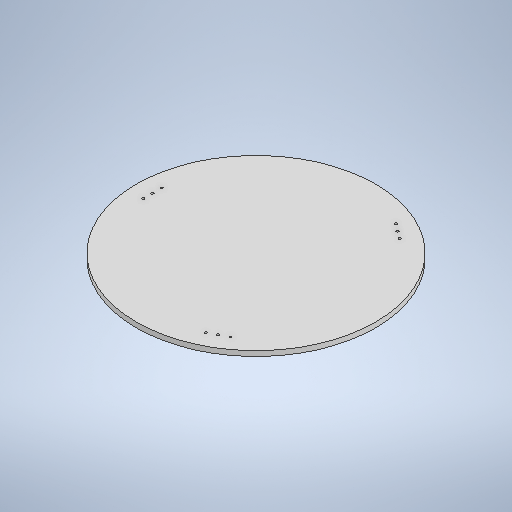
# Autodesk Inventor part: plate support
Saved by Autodesk Inventor 2025.1 (Build 291241000, 241)
## iProperties
Created: 2024-10-31
Part Number: plate support
Material: Generic
Document SubType Name: Modeling
Designer: xingj
Density: 1 g/cm^3
Appearance: Default
Author: xingj
Autodesk Inventor part; units mm, degrees
ref_plane "YZ Plane" through (0, 0, 0) normal (1, 0, 0) x (0, 1, 0)
ref_plane "XZ Plane" through (0, 0, 0) normal (0, 1, 0) x (-1, 0, 0)
ref_plane "XY Plane" through (0, 0, 0) normal (0, 0, 1) x (1, 0, 0)
sketch "Sketch1" plane through (0, 0, 0) normal (0, 1, 0) x (-1, 0, 0)
  circle A0 centre (0, 0) radius 150
  line L0 (150, 0) -> (0, 0)
  line L1 (0, 0) -> (-75, -129.9038)
  line L2 (0, 0) -> (150, 0) construction
  line L3 (0, 0) -> (-75, 129.9038)
  line L4 (0, 0) -> (150, 0) construction
  line L5 (-75, 129.9038) -> (-74.5, 129.0378)
  line L6 (-74.5, 129.0378) -> (-69.335, 120.0917)
  line L7 (-75, 129.9038) -> (-64.967, 112.5261)
  circle A1 centre (-64.967, 112.5261) radius 1.5
  line L8 (150, 0) -> (129.934, 0)
  circle A2 centre (129.934, 0) radius 1.5
  line L9 (-75, -129.9038) -> (-64.967, -112.5261)
  circle A3 centre (-64.967, -112.5261) radius 1.5
  dimension "d20" = 300
  dimension "d22" = 120
  dimension "d23" = 120
  dimension "d24" = 1
  dimension "d25" = 10.33
  dimension "d26" = 20.066
  dimension "d27" = 3
  dimension "d28" = 20.066
  dimension "d29" = 3
  dimension "d30" = 20.066
  dimension "d31" = 3
  constraints: 20 end point, 5 coincident, 5 point on line, 4 centre point, 3 horizontal, 3 point on circle, 2 equal length
  measures "d20" diameter of A0
  measures "d22" angle of L1 L2
  measures "d23" angle of L4 L3
  measures "d24" distance of L3.end L5.end
  measures "d25" distance of L5.end L6.end
  measures "d26" distance of L3.end L7.end
  measures "d27" diameter of A1
  measures "d28" distance of L4.end L8.end
  measures "d29" diameter of A2
  measures "d30" distance of L1.end L9.end
  measures "d31" diameter of A3
extrude "Extrusion1" add sketch "Sketch1" along normal blind 6.35 contours L0 A2 L3 A1 A0 | A0 L1 A3 L0 A2 | L3 A1 L1 A3 A0
sketch "Sketch2" plane through (0, 6.35, 0) normal (0, 1, 0) x (1, 0, 0)
  circle A0 centre (-129.934, 0) radius 1.5 projected
  line L0 (-129.934, -1.5) -> (-129.934, -11.5)
  line L1 (-129.934, 1.5) -> (-129.934, 11.5)
  circle A1 centre (-129.934, -11.5) radius 1.5
  circle A2 centre (-129.934, 11.5) radius 1.5
  circle A3 centre (64.967, -112.5261) radius 1.5 projected
  line L2 (63.6961, -113.3229) -> (54.8713, -118.0264)
  line L3 (54.8713, -118.0264) -> (66.337, -111.9154)
  line L4 (66.337, -111.9154) -> (75.1618, -107.2119)
  circle A4 centre (54.8713, -118.0264) radius 1.5
  circle A5 centre (75.1618, -107.2119) radius 1.5
  circle A6 centre (64.967, 112.5261) radius 1.5 projected
  line L5 (66.337, 111.9154) -> (74.3759, 105.9675)
  line L6 (74.3759, 105.9675) -> (63.9823, 113.6576)
  line L7 (63.9823, 113.6576) -> (55.9434, 119.6055)
  circle A7 centre (55.9434, 119.6055) radius 1.5
  circle A8 centre (74.3759, 105.9675) radius 1.5
  point P0 (0, 0)
  dimension "d36" = 10
  dimension "d37" = 10
  dimension "d38" = 3
  dimension "d39" = 3
  dimension "d40" = 10
  dimension "d41" = 10
  dimension "d42" = 3
  dimension "d43" = 3
  dimension "d44" = 10
  dimension "d45" = 10
  dimension "d46" = 3
  dimension "d47" = 3
  constraints: 16 end point, 6 centre point, 6 coincident, 6 point on circle, 2 vertical, 1 point on line
  measures "d36" distance of L0.start L0.end
  measures "d37" distance of L1.start L1.end
  measures "d38" diameter of A1
  measures "d39" diameter of A2
  measures "d40" distance of L2.start L2.end
  measures "d41" distance of L3.end L4.end
  measures "d42" diameter of A4
  measures "d43" diameter of A5
  measures "d44" distance of L5.start L5.end
  measures "d45" distance of L6.end L7.end
  measures "d46" diameter of A7
  measures "d47" diameter of A8
extrude "Extrusion3" cut sketch "Sketch2" against normal through all contours A1 | A2 | A4 | A5 | A7 | A8
sketch "Sketch7" plane through (0, 6.35, 0) normal (0, 1, 0) x (1, 0, 0)
  circle A0 centre (0, 0) radius 150 projected
  line L0 (150, 0) -> (-150, 0)
  constraints: 2 end point, 2 point on circle, 1 horizontal
body "Solid1"
